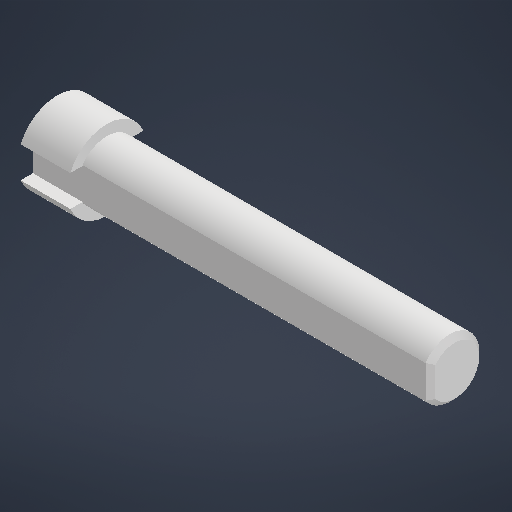
# Autodesk Inventor part: Ø6x40Shaft_Modified
Saved by Autodesk Inventor 2026 (Build 300175050, 175E)
## iProperties
Created: 2026-05-02
Part Number: Ø6x40Shaft_Modified
Material: Generic
Document SubType Name: Modeling
Designer: frede
Density: 1 g/cm^3
Appearance: Default
Author: frede
Autodesk Inventor part; units mm, degrees
ref_plane "YZ Plane" through (0, 0, 0) normal (1, 0, 0) x (0, 1, 0)
ref_plane "XZ Plane" through (0, 0, 0) normal (0, 1, 0) x (-1, 0, 0)
ref_plane "XY Plane" through (0, 0, 0) normal (0, 0, 1) x (1, 0, 0)
sketch "Sketch1" plane through (0, 0, 0) normal (1, 0, 0) x (0, 1, 0)
  circle A0 centre (0, 0) radius 2.95
  line L0 (1.6432, 2.45) -> (-1.6432, 2.45)
  dimension "d0" = 5.9
  dimension "d1" = 0.5
  constraints: 2 end point, 2 point on circle, 1 centre point, 1 coincident, 1 horizontal
  measures "d0" diameter of A0
  measures "d1" distance edge to line of A0 L0
extrude "Extrusion1" add sketch "Sketch1" along normal blind 40 contours A0 L0 picked at (0.5577, 0.5097)
chamfer "Chamfer1" distance 0.5 angle 45 4 edges at (0, 0, -2.95) (0, 0, 2.45) (40, 0, -2.95) (40, 0, 2.45)
sketch "Sketch2" plane through (0, 0, 0) normal (-1, 0, 0) x (0, 0, 1)
  circle A0 centre (0, 0) radius 3
  circle A1 centre (0, 0) radius 4
  line L0 (5.565, 1.565) -> (2.435, 1.565)
  line L1 (2.435, 1.565) -> (2.435, -1.565)
  line L2 (2.435, -1.565) -> (5.565, -1.565)
  line L3 (5.565, -1.565) -> (5.565, 1.565)
  line L4 (5.565, 1.565) -> (2.435, -1.565) construction
  line L5 (2.435, 1.565) -> (5.565, -1.565) construction
  line L6 (-2.425, 1.575) -> (-5.575, 1.575)
  line L7 (-5.575, 1.575) -> (-5.575, -1.575)
  line L8 (-5.575, -1.575) -> (-2.425, -1.575)
  line L9 (-2.425, -1.575) -> (-2.425, 1.575)
  line L10 (-2.425, 1.575) -> (-5.575, -1.575) construction
  line L11 (-5.575, 1.575) -> (-2.425, -1.575) construction
  point P0 (4, 0)
  point P1 (-4, 0)
  point P2 (-3.6769, 1.575)
  point P3 (-3.6769, -1.575)
  point P4 (3.6811, -1.565)
  point P5 (3.6811, 1.565)
  dimension "d7" = 3.13
  dimension "d8" = 3.13
  dimension "d9" = 3.15
  dimension "d10" = 3.15
  constraints: 24 end point, 4 midpoint, 4 parallel, 2 coincident, 2 horizontal, 2 perpendicular, 1 centre point, 3 other
  measures "d7" distance of L2.end L1.end
  measures "d8" distance of L1.end L0.end
  measures "d9" distance of L8.end L7.end
  measures "d10" distance of L7.end L6.end
extrude "Extrusion2" add sketch "Sketch2" against normal blind 5 contours L0 L1 L2 A0 L8 L9 L6 | A0 L6 A1 L0 | L2 A1 L8 A0
body "Solid1"
